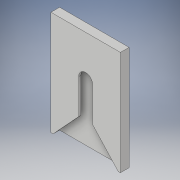
# Autodesk Inventor part: Part18
Saved by Autodesk Inventor 2019 (Build 230136000, 136)
## iProperties
Created: 2018-11-11
Part Number: Part18
Material: Generic
Document SubType Name: Modeling
Designer: maste
Density: 1 g/cm^3
Appearance: Default
Author: maste
Autodesk Inventor part; units mm, degrees
ref_plane "YZ Plane" through (0, 0, 0) normal (1, 0, 0) x (0, 1, 0)
ref_plane "XZ Plane" through (0, 0, 0) normal (0, 1, 0) x (-1, 0, 0)
ref_plane "XY Plane" through (0, 0, 0) normal (0, 0, 1) x (1, 0, 0)
sketch "Sketch1" plane through (0, 0, 0) normal (0, 0, 1) x (1, 0, 0)
  line L0 (0, 0) -> (50.8, 0)
  line L1 (50.8, 0) -> (50.8, 76.2)
  line L2 (50.8, 76.2) -> (0, 76.2)
  line L3 (0, 76.2) -> (0, 0)
  dimension "d0" = 50.8
  dimension "d1" = 76.2
  constraints: 8 end point, 2 parallel, 1 horizontal, 1 perpendicular
  measures "d0" distance of L2.end L1.end
  measures "d1" distance of L1.end L0.end
extrude "Extrusion1" add sketch "Sketch1" along normal blind 6.35
sketch "Sketch2" plane through (0, 0, 0) normal (0, -1, 0) x (1, 0, 0)
  line L0 (0, 0) -> (50.8, 0) projected
  line L1 (0, 6.35) -> (50.8, 6.35) projected
  line L2 (0, 0) -> (50.8, 0)
  line L3 (50.8, 0) -> (50.8, 6.35)
  line L4 (50.8, 6.35) -> (0, 6.35)
  line L5 (0, 6.35) -> (0, 0)
  line L6 (49.2125, 4.7625) -> (49.2125, 1.5875)
  line L7 (49.2125, 1.5875) -> (1.5875, 1.5875)
  line L8 (1.5875, 1.5875) -> (1.5875, 4.7625)
  line L9 (1.5875, 4.7625) -> (49.2125, 4.7625)
  dimension "d4" = 1.5875
  constraints: 16 end point, 4 parallel, 2 perpendicular, 1 horizontal, 3 other
  measures "d4" distance between parallel lines of L3 L6
extrude "Extrusion2" cut sketch "Sketch2" against normal blind 63.5 contours L6 L7 L8 L9
sketch "Sketch3" plane through (0, 0, 6.35) normal (0, 0, 1) x (1, 0, 0)
  line L0 (50.8, 76.2) -> (0, 76.2) projected
  line L1 (25.4, 76.2) -> (25.4, 0)
  line L2 (49.2125, 0) -> (1.5875, 0) projected
  line L3 (30.48, 76.2) -> (30.48, 0)
  line L4 (20.32, 76.2) -> (20.32, 0)
  line L5 (49.2125, 63.5) -> (1.5875, 63.5) projected
  line L6 (25.4, 63.5) -> (25.4, 50.8)
  line L7 (25.4, 50.8) -> (25.4, 45.72)
  circle A0 centre (25.4, 45.72) radius 5.08
  line L8 (30.48, 45.72) -> (30.48, 20.32)
  line L9 (49.2125, 0) -> (49.2125, 63.5) projected
  line L10 (30.48, 20.32) -> (49.2125, 0)
  line L11 (20.32, 45.72) -> (20.32, 20.32)
  line L12 (20.32, 20.32) -> (1.5875, 0)
  point P0 (0, 0)
  dimension "d7" = 5.08
  dimension "d8" = 5.08
  dimension "d9" = 12.7
  dimension "d10" = 5.08
  dimension "d11" = 25.4
  dimension "d12" = 25.4
  constraints: 18 end point, 6 point on line, 3 midpoint, 3 point on circle, 2 parallel, 1 centre point, 1 coincident
  measures "d7" distance between parallel lines of L1 L3
  measures "d8" distance between parallel lines of L1 L4
  measures "d9" distance of L6.start L6.end
  measures "d10" distance of L6.end L7.end
  measures "d11" distance of L8.start L8.end
  measures "d12" distance of L11.start L11.end
extrude "Extrusion3" cut sketch "Sketch3" against normal blind 4.7625 contours A0 L1 | L3 L2 L1 A0 | L1 A0 | L10 L2 L3 | L1 L2 L4 A0 | L4 L2 L12
body "Solid1"
